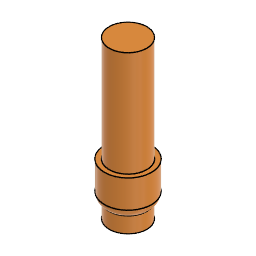
PropellerStand (Autodesk Fusion 360 design; units mm, degrees)
part number: 2026-06-05-00-18-02-927
Autodesk Fusion 360 part; units mm, degrees
sketch "Sketch1" plane through (0, 0, 0) normal (0, 0, 1) x (1, 0, 0)
  circle A0 centre (0, 0) radius 1.2
  circle A1 centre (0, 0) radius 1.5
  dimension "d1" = 2.4
  dimension "d2" = 3
  constraint coincident A0.centre A1.centre
  constraint concentric A0 A1
  measures "d1" diameter of A0
  measures "d2" diameter of A1
extrude "Extrude2" add sketch "Sketch1" along normal blind 2.3 from surface at 1 contours A0 | A1
extrude "Extrude3" add sketch "Sketch1" along normal blind 10 contours A0
fillet "Fillet1" radius 0.6 1 edges at (-1.3985, -0.5424, 1)
named bodies: "Body1"
